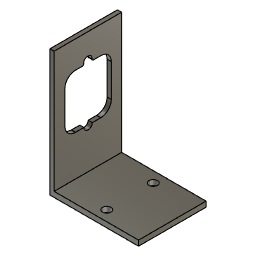
camera_support_angle_v4 (Autodesk Fusion 360 design; units mm, degrees)
Autodesk Fusion 360 part; units mm, degrees
sketch "Sketch1" plane through (0, 0, 0) normal (0, 0, 1) x (1, 0, 0)
  line L0 (-30.0236, 16) -> (9.9764, 16)
  line L1 (9.9764, 16) -> (9.9764, -16)
  line L2 (9.9764, -16) -> (-30.0236, -16)
  line L3 (-30.0236, -16) -> (-30.0236, 16)
  line L4 (-32, 16) -> (-30.0236, 16)
  line L5 (-30.0236, 16) -> (-30.0236, -16)
  line L6 (-30.0236, -16) -> (-32, -16)
  line L7 (-32, -16) -> (-32, 16)
  circle A0 centre (-5.1148, 11.0232) radius 2
  circle A1 centre (-5.0484, -11.0135) radius 2
  line L8 (-0.0236, 28) -> (-0.0236, -28) construction
  circle A2 through (77, 11, 2.5) (74, 12.7321, 2.5) (74, 9.2679, 2.5)
  circle A3 through (77, -11, 2.5) (74, -9.2679, 2.5) (74, -12.7321, 2.5)
  line L9 (-36, 11) -> (79, 11) construction
  line L10 (-36, -11) -> (79, -11) construction
  dimension "d1" = 40
  dimension "d2" = 4
  dimension "d5" = 4
  dimension "d45" = 30
  constraint vertical L1
  constraint horizontal L2
  constraint vertical L3
  constraint vertical L5
  constraint vertical L7
  constraint perpendicular L0 L8
  constraint perpendicular L8 L9
  constraint perpendicular L7 L10
  measures "d1" distance of L1.end L2.end
  measures "d2" diameter of A0
  measures "d5" diameter of A1
  measures "d45" distance of L5 L8
extrude "Extrude1" add sketch "Sketch1" along normal blind 2.5
extrude "Extrude2" add sketch "Sketch1" along normal blind 60 contours L3 L4 L5 L6 L7
sketch "Sketch2" plane through (0, 0, 0) normal (1, 0, 0) x (0, 1, 0)
  line L0 (0.1131, -9) -> (0.1131, 42.4658) construction
  line L1 (16.5, 8.5) -> (-22, 8.5) construction
  line L2 (20, 35.1684) -> (-25, 35.1684)
  line L3 (19, 5) -> (-25, 5) construction
  line L4 (11.1131, -9) -> (11.1131, 42.4658) construction
  line L5 (-10.8869, -9) -> (-10.8869, 42.1284) construction
  line L6 (-2.4755, 47.1284) -> (-5.8869, 47.1284)
  line L7 (-10.8868, 47.5935) -> (-10.8868, 26.6406)
  line L8 (-5.8868, 21.6406) -> (6.113, 21.6406)
  line L9 (11.113, 26.6406) -> (11.113, 42.1284)
  arc A0 (11.113, 42.1284) -> (6.113, 47.1284) centre (6.113, 42.1284) ccw
  arc A1 (6.113, 21.6406) -> (11.113, 26.6406) centre (6.113, 26.6406) ccw
  arc A2 (-10.8868, 26.6406) -> (-5.8868, 21.6406) centre (-5.8868, 26.6406) ccw
  arc A3 (-5.8869, 47.1284) -> (-10.8869, 42.1284) centre (-5.8869, 42.1284) ccw
  circle A4 centre (0.1131, 21.6406) radius 2
  line L10 (-14, 0) -> (32, 0) construction
  arc A5 (1.9721, 47.7045) -> (-1.9813, 47.7045) centre (-0.0046, 48.009) ccw
  arc A6 (-2.4755, 47.1284) -> (-1.9813, 47.7045) centre (-2.4755, 47.6284) ccw
  line L11 (6.113, 47.1284) -> (2.4662, 47.1284)
  arc A7 (1.9721, 47.7045) -> (2.4662, 47.1284) centre (2.4662, 47.6284) ccw
  dimension "d10" = 11
  dimension "d13" = 5
  dimension "d16" = 5
  dimension "d40" = 4
  dimension "d48" = 11.9998
  dimension "d50" = 0.5
  dimension "d51" = 0.5
  constraint vertical L0
  constraint horizontal L1
  constraint perpendicular L0 L2
  constraint parallel L1 L3
  constraint horizontal L6
  constraint vertical L7
  constraint horizontal L8
  constraint vertical L9
  constraint tangent L6 A0
  constraint tangent L9 A0
  constraint tangent L8 A1
  constraint tangent L9 A1
  constraint equal A0 A1
  constraint tangent L7 A2
  constraint tangent L8 A2
  constraint equal A0 A2
  constraint tangent L6 A3
  constraint tangent L5 A3
  constraint midpoint L8 A4.centre
  constraint perpendicular L5 L10
  constraint tangent A5 A6
  constraint tangent L6 A6
  constraint tangent A0 L11
  constraint tangent L11 A7
  constraint tangent A5 A7
  measures "d13" radius of A0
  measures "d16" radius of A3
  measures "d40" diameter of A4
  measures "d48" distance of L8.end L8.start
  measures "d50" radius of A6
  measures "d51" radius of A7
extrude "Extrude3" cut sketch "Sketch2" against normal blind 45 contours L2 L7 L8 L9 A1 A2 A4 | L2 L6 L7 L9 A0 A3 A5 A6 L11 A7 | L8 A4 picked at (0.6018, 22.094)
sketch "Sketch3" plane through (0, 0, 2.5) normal (0, 0, 1) x (-1, 0, 0)
  line L0 (30.0236, -16) -> (30.0236, 16)
  line L1 (30.0236, 16) -> (-9.9764, 16)
  line L2 (-9.9764, 16) -> (-9.9764, -16)
  line L3 (-9.9764, -16) -> (30.0236, -16)
  circle A0 centre (5.1148, -11.0232) radius 2
  circle A1 centre (5.0484, 11.0135) radius 2
  line L4 (-9.9764, 16) -> (-9.9764, -16)
  constraint vertical L4
  constraint coincident L2.end L3.start
extrude "Extrude4" add sketch "Sketch3" against normal blind 2.5 contours L0 L1 L2 L3 L4 | A0 | A1
hole "Hole2" at (75, 11, 2.5) direction (0, 0, -1) diameter 4 depth 40 tip angle 180
hole "Hole3" at (75, -11, 2.5) direction (0, 0, -1) diameter 4 depth 40 tip angle 180
hole "Hole4" at (-9.9934, 10.9168, 2.5) direction (0, 0, -1) diameter 4 depth 40 tip angle 180
hole "Hole5" at (-10.0059, -11.0767, 2.5) direction (0, 0, -1) diameter 4 depth 40 tip angle 180
extrude "Extrude6" cut sketch "Sketch2" against normal blind 80 contours L2 L6 L7 L9 A0 A3 A5 A6 L11 A7 | L8 A4 picked at (-0.3756, 21.1871)
extrude "Extrude5" [suppressed]
